Autodesk Fusion 360 part; units mm, degrees
(part 3 of 40)
  spline S12 degree 5 poles (236.3268, 206.0345) (236.3391, 206.0628) (236.3628, 206.1198) (236.396, 206.2062) (236.4359, 206.3229) (236.4798, 206.4711) (236.5193, 206.6208) (236.5561, 206.7714) (236.5915, 206.9226) (236.626, 207.0741) (236.6594, 207.226) (236.6914, 207.3783) (236.7216, 207.5312) (236.7496, 207.6848) (236.7755, 207.8391) (236.7994, 207.994) (236.8217, 208.1494) (236.8425, 208.3052) (236.8621, 208.4614) (236.8805, 208.6179) (236.8978, 208.7747) (236.9138, 208.9318) (236.9285, 209.0893) (236.9418, 209.2471) (236.9538, 209.4053) (236.9645, 209.5638) (236.974, 209.7226) (236.9824, 209.8817) (236.9897, 210.0411) (236.9958, 210.2007) (237.0009, 210.3605) (237.0049, 210.5206) (237.0077, 210.6809) (237.0096, 210.8415) (237.0103, 211.0023) (237.01, 211.1633) (237.0086, 211.3245) (237.0062, 211.4859) (237.0028, 211.6475) (236.9985, 211.8093) (236.9931, 211.9712) (236.9868, 212.1334) (236.9795, 212.2957) (236.9712, 212.4581) (236.962, 212.6207) (236.9519, 212.7835) (236.9408, 212.9464) (236.9287, 213.1095) (236.9158, 213.2727) (236.902, 213.436) (236.8872, 213.5995) (236.8716, 213.7631) (236.855, 213.9268) (236.8376, 214.0906) (236.8193, 214.2545) (236.8001, 214.4185) (236.78, 214.5826) (236.7591, 214.7468) (236.7374, 214.9111) (236.7148, 215.0755) (236.6913, 215.24) (236.667, 215.4046) (236.6418, 215.5692) (236.6159, 215.734) (236.5891, 215.8987) (236.5614, 216.0636) (236.533, 216.2285) (236.5038, 216.3935) (236.4737, 216.5585) (236.4428, 216.7236) (236.4112, 216.8887) (236.3852, 217.0208) (236.3654, 217.1199) (236.352, 217.186) (236.3452, 217.2191) knots 0 0 0 0 0 0 0.01428571 0.02857143 0.04285714 0.05714286 0.07142857 0.08571429 0.1 0.11428571 0.12857143 0.14285714 0.15714286 0.17142857 0.18571429 0.2 0.21428571 0.22857143 0.24285714 0.25714286 0.27142857 0.28571429 0.3 0.31428571 0.32857143 0.34285714 0.35714286 0.37142857 0.38571429 0.4 0.41428571 0.42857143 0.44285714 0.45714286 0.47142857 0.48571429 0.5 0.51428571 0.52857143 0.54285714 0.55714286 0.57142857 0.58571429 0.6 0.61428571 0.62857143 0.64285714 0.65714286 0.67142857 0.68571429 0.7 0.71428571 0.72857143 0.74285714 0.75714286 0.77142857 0.78571429 0.8 0.81428571 0.82857143 0.84285714 0.85714286 0.87142857 0.88571429 0.9 0.91428571 0.92857143 0.94285714 0.95714286 0.97142857 0.98571429 1 1 1 1 1 1
  line L899 (236.3268, 206.0345) -> (236.3391, 206.0628) construction
  line L900 (236.3391, 206.0628) -> (236.3628, 206.1198) construction
  line L901 (236.3628, 206.1198) -> (236.396, 206.2062) construction
  line L902 (236.396, 206.2062) -> (236.4359, 206.3229) construction
  line L903 (236.4359, 206.3229) -> (236.4798, 206.4711) construction
  line L904 (236.4798, 206.4711) -> (236.5193, 206.6208) construction
  line L905 (236.5193, 206.6208) -> (236.5561, 206.7714) construction
  line L906 (236.5561, 206.7714) -> (236.5915, 206.9226) construction
  line L907 (236.5915, 206.9226) -> (236.626, 207.0741) construction
  line L908 (236.626, 207.0741) -> (236.6594, 207.226) construction
  line L909 (236.6594, 207.226) -> (236.6914, 207.3783) construction
  line L910 (236.6914, 207.3783) -> (236.7216, 207.5312) construction
  line L911 (236.7216, 207.5312) -> (236.7496, 207.6848) construction
  line L912 (236.7496, 207.6848) -> (236.7755, 207.8391) construction
  line L913 (236.7755, 207.8391) -> (236.7994, 207.994) construction
  line L914 (236.7994, 207.994) -> (236.8217, 208.1494) construction
  line L915 (236.8217, 208.1494) -> (236.8425, 208.3052) construction
  line L916 (236.8425, 208.3052) -> (236.8621, 208.4614) construction
  line L917 (236.8621, 208.4614) -> (236.8805, 208.6179) construction
  line L918 (236.8805, 208.6179) -> (236.8978, 208.7747) construction
  line L919 (236.8978, 208.7747) -> (236.9138, 208.9318) construction
  line L920 (236.9138, 208.9318) -> (236.9285, 209.0893) construction
  line L921 (236.9285, 209.0893) -> (236.9418, 209.2471) construction
  line L922 (236.9418, 209.2471) -> (236.9538, 209.4053) construction
  line L923 (236.9538, 209.4053) -> (236.9645, 209.5638) construction
  line L924 (236.9645, 209.5638) -> (236.974, 209.7226) construction
  line L925 (236.974, 209.7226) -> (236.9824, 209.8817) construction
  line L926 (236.9824, 209.8817) -> (236.9897, 210.0411) construction
  line L927 (236.9897, 210.0411) -> (236.9958, 210.2007) construction
  line L928 (236.9958, 210.2007) -> (237.0009, 210.3605) construction
  line L929 (237.0009, 210.3605) -> (237.0049, 210.5206) construction
  line L930 (237.0049, 210.5206) -> (237.0077, 210.6809) construction
  line L931 (237.0077, 210.6809) -> (237.0096, 210.8415) construction
  line L932 (237.0096, 210.8415) -> (237.0103, 211.0023) construction
  line L933 (237.0103, 211.0023) -> (237.01, 211.1633) construction
  line L934 (237.01, 211.1633) -> (237.0086, 211.3245) construction
  line L935 (237.0086, 211.3245) -> (237.0062, 211.4859) construction
  line L936 (237.0062, 211.4859) -> (237.0028, 211.6475) construction
  line L937 (237.0028, 211.6475) -> (236.9985, 211.8093) construction
  line L938 (236.9985, 211.8093) -> (236.9931, 211.9712) construction
  line L939 (236.9931, 211.9712) -> (236.9868, 212.1334) construction
  line L940 (236.9868, 212.1334) -> (236.9795, 212.2957) construction
  line L941 (236.9795, 212.2957) -> (236.9712, 212.4581) construction
  line L942 (236.9712, 212.4581) -> (236.962, 212.6207) construction
  line L943 (236.962, 212.6207) -> (236.9519, 212.7835) construction
  line L944 (236.9519, 212.7835) -> (236.9408, 212.9464) construction
  line L945 (236.9408, 212.9464) -> (236.9287, 213.1095) construction
  line L946 (236.9287, 213.1095) -> (236.9158, 213.2727) construction
  line L947 (236.9158, 213.2727) -> (236.902, 213.436) construction
  line L948 (236.902, 213.436) -> (236.8872, 213.5995) construction
  line L949 (236.8872, 213.5995) -> (236.8716, 213.7631) construction
  line L950 (236.8716, 213.7631) -> (236.855, 213.9268) construction
  line L951 (236.855, 213.9268) -> (236.8376, 214.0906) construction
  line L952 (236.8376, 214.0906) -> (236.8193, 214.2545) construction
  line L953 (236.8193, 214.2545) -> (236.8001, 214.4185) construction
  line L954 (236.8001, 214.4185) -> (236.78, 214.5826) construction
  line L955 (236.78, 214.5826) -> (236.7591, 214.7468) construction
  line L956 (236.7591, 214.7468) -> (236.7374, 214.9111) construction
  line L957 (236.7374, 214.9111) -> (236.7148, 215.0755) construction
  line L958 (236.7148, 215.0755) -> (236.6913, 215.24) construction
  line L959 (236.6913, 215.24) -> (236.667, 215.4046) construction
  line L960 (236.667, 215.4046) -> (236.6418, 215.5692) construction
  line L961 (236.6418, 215.5692) -> (236.6159, 215.734) construction
  line L962 (236.6159, 215.734) -> (236.5891, 215.8987) construction
  line L963 (236.5891, 215.8987) -> (236.5614, 216.0636) construction
  line L964 (236.5614, 216.0636) -> (236.533, 216.2285) construction
  line L965 (236.533, 216.2285) -> (236.5038, 216.3935) construction
  line L966 (236.5038, 216.3935) -> (236.4737, 216.5585) construction
  line L967 (236.4737, 216.5585) -> (236.4428, 216.7236) construction
  line L968 (236.4428, 216.7236) -> (236.4112, 216.8887) construction
  line L969 (236.4112, 216.8887) -> (236.3852, 217.0208) construction
  line L970 (236.3852, 217.0208) -> (236.3654, 217.1199) construction
  line L971 (236.3654, 217.1199) -> (236.352, 217.186) construction
  line L972 (236.352, 217.186) -> (236.3452, 217.2191) construction
  spline S13 degree 5 poles (236.3268, 206.0345) (236.3391, 206.0628) (236.3628, 206.1198) (236.396, 206.2062) (236.4359, 206.3229) (236.4798, 206.4711) (236.5193, 206.6208) (236.5561, 206.7714) (236.5915, 206.9226) (236.626, 207.0741) (236.6594, 207.226) (236.6914, 207.3783) (236.7216, 207.5312) (236.7496, 207.6848) (236.7755, 207.8391) (236.7994, 207.994) (236.8217, 208.1494) (236.8425, 208.3052) (236.8621, 208.4614) (236.8805, 208.6179) (236.8978, 208.7747) (236.9138, 208.9318) (236.9285, 209.0893) (236.9418, 209.2471) (236.9538, 209.4053) (236.9645, 209.5638) (236.974, 209.7226) (236.9824, 209.8817) (236.9897, 210.0411) (236.9958, 210.2007) (237.0009, 210.3605) (237.0049, 210.5206) (237.0077, 210.6809) (237.0096, 210.8415) (237.0103, 211.0023) (237.01, 211.1633) (237.0086, 211.3245) (237.0062, 211.4859) (237.0028, 211.6475) (236.9985, 211.8093) (236.9931, 211.9712) (236.9868, 212.1334) (236.9795, 212.2957) (236.9712, 212.4581) (236.962, 212.6207) (236.9519, 212.7835) (236.9408, 212.9464) (236.9287, 213.1095) (236.9158, 213.2727) (236.902, 213.436) (236.8872, 213.5995) (236.8716, 213.7631) (236.855, 213.9268) (236.8376, 214.0906) (236.8193, 214.2545) (236.8001, 214.4185) (236.78, 214.5826) (236.7591, 214.7468) (236.7374, 214.9111) (236.7148, 215.0755) (236.6913, 215.24) (236.667, 215.4046) (236.6418, 215.5692) (236.6159, 215.734) (236.5891, 215.8987) (236.5614, 216.0636) (236.533, 216.2285) (236.5038, 216.3935) (236.4737, 216.5585) (236.4428, 216.7236) (236.4112, 216.8887) (236.3852, 217.0208) (236.3654, 217.1199) (236.352, 217.186) (236.3452, 217.2191) knots 0 0 0 0 0 0 0.01428571 0.02857143 0.04285714 0.05714286 0.07142857 0.08571429 0.1 0.11428571 0.12857143 0.14285714 0.15714286 0.17142857 0.18571429 0.2 0.21428571 0.22857143 0.24285714 0.25714286 0.27142857 0.28571429 0.3 0.31428571 0.32857143 0.34285714 0.35714286 0.37142857 0.38571429 0.4 0.41428571 0.42857143 0.44285714 0.45714286 0.47142857 0.48571429 0.5 0.51428571 0.52857143 0.54285714 0.55714286 0.57142857 0.58571429 0.6 0.61428571 0.62857143 0.64285714 0.65714286 0.67142857 0.68571429 0.7 0.71428571 0.72857143 0.74285714 0.75714286 0.77142857 0.78571429 0.8 0.81428571 0.82857143 0.84285714 0.85714286 0.87142857 0.88571429 0.9 0.91428571 0.92857143 0.94285714 0.95714286 0.97142857 0.98571429 1 1 1 1 1 1
  line L973 (236.3268, 206.0345) -> (236.3391, 206.0628) construction
  line L974 (236.3391, 206.0628) -> (236.3628, 206.1198) construction
  line L975 (236.3628, 206.1198) -> (236.396, 206.2062) construction
  line L976 (236.396, 206.2062) -> (236.4359, 206.3229) construction
  line L977 (236.4359, 206.3229) -> (236.4798, 206.4711) construction
  line L978 (236.4798, 206.4711) -> (236.5193, 206.6208) construction
  line L979 (236.5193, 206.6208) -> (236.5561, 206.7714) construction
  line L980 (236.5561, 206.7714) -> (236.5915, 206.9226) construction
  line L981 (236.5915, 206.9226) -> (236.626, 207.0741) construction
  line L982 (236.626, 207.0741) -> (236.6594, 207.226) construction
  line L983 (236.6594, 207.226) -> (236.6914, 207.3783) construction
  line L984 (236.6914, 207.3783) -> (236.7216, 207.5312) construction
  line L985 (236.7216, 207.5312) -> (236.7496, 207.6848) construction
  line L986 (236.7496, 207.6848) -> (236.7755, 207.8391) construction
  line L987 (236.7755, 207.8391) -> (236.7994, 207.994) construction
  line L988 (236.7994, 207.994) -> (236.8217, 208.1494) construction
  line L989 (236.8217, 208.1494) -> (236.8425, 208.3052) construction
  line L990 (236.8425, 208.3052) -> (236.8621, 208.4614) construction
  line L991 (236.8621, 208.4614) -> (236.8805, 208.6179) construction
  line L992 (236.8805, 208.6179) -> (236.8978, 208.7747) construction
  line L993 (236.8978, 208.7747) -> (236.9138, 208.9318) construction
  line L994 (236.9138, 208.9318) -> (236.9285, 209.0893) construction
  line L995 (236.9285, 209.0893) -> (236.9418, 209.2471) construction
  line L996 (236.9418, 209.2471) -> (236.9538, 209.4053) construction
  line L997 (236.9538, 209.4053) -> (236.9645, 209.5638) construction
  line L998 (236.9645, 209.5638) -> (236.974, 209.7226) construction
  line L999 (236.974, 209.7226) -> (236.9824, 209.8817) construction
  line L1000 (236.9824, 209.8817) -> (236.9897, 210.0411) construction
  line L1001 (236.9897, 210.0411) -> (236.9958, 210.2007) construction
  line L1002 (236.9958, 210.2007) -> (237.0009, 210.3605) construction
  line L1003 (237.0009, 210.3605) -> (237.0049, 210.5206) construction
  line L1004 (237.0049, 210.5206) -> (237.0077, 210.6809) construction
  line L1005 (237.0077, 210.6809) -> (237.0096, 210.8415) construction
  line L1006 (237.0096, 210.8415) -> (237.0103, 211.0023) construction
  line L1007 (237.0103, 211.0023) -> (237.01, 211.1633) construction
  line L1008 (237.01, 211.1633) -> (237.0086, 211.3245) construction
  line L1009 (237.0086, 211.3245) -> (237.0062, 211.4859) construction
  line L1010 (237.0062, 211.4859) -> (237.0028, 211.6475) construction
  line L1011 (237.0028, 211.6475) -> (236.9985, 211.8093) construction
  line L1012 (236.9985, 211.8093) -> (236.9931, 211.9712) construction
  line L1013 (236.9931, 211.9712) -> (236.9868, 212.1334) construction
  line L1014 (236.9868, 212.1334) -> (236.9795, 212.2957) construction
  line L1015 (236.9795, 212.2957) -> (236.9712, 212.4581) construction
  line L1016 (236.9712, 212.4581) -> (236.962, 212.6207) construction
  line L1017 (236.962, 212.6207) -> (236.9519, 212.7835) construction
  line L1018 (236.9519, 212.7835) -> (236.9408, 212.9464) construction
  line L1019 (236.9408, 212.9464) -> (236.9287, 213.1095) construction
  line L1020 (236.9287, 213.1095) -> (236.9158, 213.2727) construction
  line L1021 (236.9158, 213.2727) -> (236.902, 213.436) construction
  line L1022 (236.902, 213.436) -> (236.8872, 213.5995) construction
  line L1023 (236.8872, 213.5995) -> (236.8716, 213.7631) construction
  line L1024 (236.8716, 213.7631) -> (236.855, 213.9268) construction
  line L1025 (236.855, 213.9268) -> (236.8376, 214.0906) construction
  line L1026 (236.8376, 214.0906) -> (236.8193, 214.2545) construction
  line L1027 (236.8193, 214.2545) -> (236.8001, 214.4185) construction
  line L1028 (236.8001, 214.4185) -> (236.78, 214.5826) construction
  line L1029 (236.78, 214.5826) -> (236.7591, 214.7468) construction
  line L1030 (236.7591, 214.7468) -> (236.7374, 214.9111) construction
  line L1031 (236.7374, 214.9111) -> (236.7148, 215.0755) construction
  line L1032 (236.7148, 215.0755) -> (236.6913, 215.24) construction
  line L1033 (236.6913, 215.24) -> (236.667, 215.4046) construction
  line L1034 (236.667, 215.4046) -> (236.6418, 215.5692) construction
  line L1035 (236.6418, 215.5692) -> (236.6159, 215.734) construction
  line L1036 (236.6159, 215.734) -> (236.5891, 215.8987) construction
  line L1037 (236.5891, 215.8987) -> (236.5614, 216.0636) construction
  line L1038 (236.5614, 216.0636) -> (236.533, 216.2285) construction
  line L1039 (236.533, 216.2285) -> (236.5038, 216.3935) construction
  line L1040 (236.5038, 216.3935) -> (236.4737, 216.5585) construction
  line L1041 (236.4737, 216.5585) -> (236.4428, 216.7236) construction
  line L1042 (236.4428, 216.7236) -> (236.4112, 216.8887) construction
  line L1043 (236.4112, 216.8887) -> (236.3852, 217.0208) construction
  line L1044 (236.3852, 217.0208) -> (236.3654, 217.1199) construction
  line L1045 (236.3654, 217.1199) -> (236.352, 217.186) construction
  line L1046 (236.352, 217.186) -> (236.3452, 217.2191) construction
  line L1047 (167.5414, 110.7517) -> (166.3167, 109.6737)
  line L1048 (167.5414, 110.7517) -> (166.3167, 109.6737)
  arc A19 (235.6801, 204.5366) -> (236.6621, 201.9354) centre (237.5162, 203.7438) ccw
  line L1049 (235.6801, 204.5366) -> (236.3268, 206.0345)
  line L1050 (235.6801, 204.5366) -> (236.3268, 206.0345)
  arc A20 (235.6801, 204.5366) -> (236.6621, 201.9354) centre (237.5162, 203.7438) ccw
  line L1051 (167.5414, 189.2483) -> (166.3167, 190.3263)
  spline S14 degree 5 poles (243.2435, 202.5103) (243.2592, 202.5368) (243.2914, 202.5895) (243.3417, 202.6672) (243.4127, 202.7681) (243.5068, 202.8906) (243.6047, 203.0106) (243.7049, 203.1289) (243.8064, 203.2464) (243.9087, 203.3634) (244.012, 203.4797) (244.1164, 203.5951) (244.2223, 203.7094) (244.3301, 203.8224) (244.4397, 203.934) (244.551, 204.0444) (244.6636, 204.1537) (244.7775, 204.2622) (244.8923, 204.3698) (245.008, 204.4767) (245.1247, 204.5828) (245.2425, 204.6881) (245.3612, 204.7926) (245.4811, 204.8961) (245.602, 204.9988) (245.7239, 205.1007) (245.8468, 205.2017) (245.9706, 205.302) (246.0953, 205.4015) (246.2208, 205.5003) (246.3471, 205.5984) (246.4743, 205.6957) (246.6023, 205.7923) (246.7311, 205.8881) (246.8608, 205.9832) (246.9912, 206.0776) (247.1225, 206.1712) (247.2544, 206.2642) (247.3872, 206.3564) (247.5206, 206.448) (247.6548, 206.5388) (247.7897, 206.629) (247.9253, 206.7185) (248.0615, 206.8073) (248.1985, 206.8955) (248.3362, 206.9829) (248.4745, 207.0697) (248.6135, 207.1558) (248.7531, 207.2413) (248.8934, 207.3261) (249.0343, 207.4102) (249.1758, 207.4937) (249.318, 207.5765) (249.4608, 207.6587) (249.6041, 207.7403) (249.7481, 207.8212) (249.8927, 207.9014) (250.0378, 207.981) (250.1835, 208.06) (250.3298, 208.1383) (250.4767, 208.216) (250.6241, 208.2931) (250.7721, 208.3695) (250.9206, 208.4453) (251.0697, 208.5205) (251.2193, 208.595) (251.3694, 208.669) (251.5201, 208.7423) (251.6713, 208.8149) (251.8229, 208.887) (251.9751, 208.9584) (252.0973, 209.0151) (252.1892, 209.0573) (252.2505, 209.0853) (252.2812, 209.0993) knots 0 0 0 0 0 0 0.01428571 0.02857143 0.04285714 0.05714286 0.07142857 0.08571429 0.1 0.11428571 0.12857143 0.14285714 0.15714286 0.17142857 0.18571429 0.2 0.21428571 0.22857143 0.24285714 0.25714286 0.27142857 0.28571429 0.3 0.31428571 0.32857143 0.34285714 0.35714286 0.37142857 0.38571429 0.4 0.41428571 0.42857143 0.44285714 0.45714286 0.47142857 0.48571429 0.5 0.51428571 0.52857143 0.54285714 0.55714286 0.57142857 0.58571429 0.6 0.61428571 0.62857143 0.64285714 0.65714286 0.67142857 0.68571429 0.7 0.71428571 0.72857143 0.74285714 0.75714286 0.77142857 0.78571429 0.8 0.81428571 0.82857143 0.84285714 0.85714286 0.87142857 0.88571429 0.9 0.91428571 0.92857143 0.94285714 0.95714286 0.97142857 0.98571429 1 1 1 1 1 1
  line L1052 (243.2435, 202.5103) -> (243.2592, 202.5368) construction
  line L1053 (243.2592, 202.5368) -> (243.2914, 202.5895) construction
  line L1054 (243.2914, 202.5895) -> (243.3417, 202.6672) construction
  line L1055 (243.3417, 202.6672) -> (243.4127, 202.7681) construction
  line L1056 (243.4127, 202.7681) -> (243.5068, 202.8906) construction
  line L1057 (243.5068, 202.8906) -> (243.6047, 203.0106) construction
  line L1058 (243.6047, 203.0106) -> (243.7049, 203.1289) construction
  line L1059 (243.7049, 203.1289) -> (243.8064, 203.2464) construction
  line L1060 (243.8064, 203.2464) -> (243.9087, 203.3634) construction
  line L1061 (243.9087, 203.3634) -> (244.012, 203.4797) construction
  line L1062 (244.012, 203.4797) -> (244.1164, 203.5951) construction
  line L1063 (244.1164, 203.5951) -> (244.2223, 203.7094) construction
  line L1064 (244.2223, 203.7094) -> (244.3301, 203.8224) construction
  line L1065 (244.3301, 203.8224) -> (244.4397, 203.934) construction
  line L1066 (244.4397, 203.934) -> (244.551, 204.0444) construction
  line L1067 (244.551, 204.0444) -> (244.6636, 204.1537) construction
  line L1068 (244.6636, 204.1537) -> (244.7775, 204.2622) construction
  line L1069 (244.7775, 204.2622) -> (244.8923, 204.3698) construction
  line L1070 (244.8923, 204.3698) -> (245.008, 204.4767) construction
  line L1071 (245.008, 204.4767) -> (245.1247, 204.5828) construction
  line L1072 (245.1247, 204.5828) -> (245.2425, 204.6881) construction
  line L1073 (245.2425, 204.6881) -> (245.3612, 204.7926) construction
  line L1074 (245.3612, 204.7926) -> (245.4811, 204.8961) construction
  line L1075 (245.4811, 204.8961) -> (245.602, 204.9988) construction
  line L1076 (245.602, 204.9988) -> (245.7239, 205.1007) construction
  line L1077 (245.7239, 205.1007) -> (245.8468, 205.2017) construction
  line L1078 (245.8468, 205.2017) -> (245.9706, 205.302) construction
  line L1079 (245.9706, 205.302) -> (246.0953, 205.4015) construction
  line L1080 (246.0953, 205.4015) -> (246.2208, 205.5003) construction
  line L1081 (246.2208, 205.5003) -> (246.3471, 205.5984) construction
  line L1082 (246.3471, 205.5984) -> (246.4743, 205.6957) construction
  line L1083 (246.4743, 205.6957) -> (246.6023, 205.7923) construction
  line L1084 (246.6023, 205.7923) -> (246.7311, 205.8881) construction
  line L1085 (246.7311, 205.8881) -> (246.8608, 205.9832) construction
  line L1086 (246.8608, 205.9832) -> (246.9912, 206.0776) construction
  line L1087 (246.9912, 206.0776) -> (247.1225, 206.1712) construction
  line L1088 (247.1225, 206.1712) -> (247.2544, 206.2642) construction
  line L1089 (247.2544, 206.2642) -> (247.3872, 206.3564) construction
  line L1090 (247.3872, 206.3564) -> (247.5206, 206.448) construction
  line L1091 (247.5206, 206.448) -> (247.6548, 206.5388) construction
  line L1092 (247.6548, 206.5388) -> (247.7897, 206.629) construction
  line L1093 (247.7897, 206.629) -> (247.9253, 206.7185) construction
  line L1094 (247.9253, 206.7185) -> (248.0615, 206.8073) construction
  line L1095 (248.0615, 206.8073) -> (248.1985, 206.8955) construction
  line L1096 (248.1985, 206.8955) -> (248.3362, 206.9829) construction
  line L1097 (248.3362, 206.9829) -> (248.4745, 207.0697) construction
  line L1098 (248.4745, 207.0697) -> (248.6135, 207.1558) construction
  line L1099 (248.6135, 207.1558) -> (248.7531, 207.2413) construction
  line L1100 (248.7531, 207.2413) -> (248.8934, 207.3261) construction
  line L1101 (248.8934, 207.3261) -> (249.0343, 207.4102) construction
  line L1102 (249.0343, 207.4102) -> (249.1758, 207.4937) construction
  line L1103 (249.1758, 207.4937) -> (249.318, 207.5765) construction
  line L1104 (249.318, 207.5765) -> (249.4608, 207.6587) construction
  line L1105 (249.4608, 207.6587) -> (249.6041, 207.7403) construction
  line L1106 (249.6041, 207.7403) -> (249.7481, 207.8212) construction
  line L1107 (249.7481, 207.8212) -> (249.8927, 207.9014) construction
  line L1108 (249.8927, 207.9014) -> (250.0378, 207.981) construction
  line L1109 (250.0378, 207.981) -> (250.1835, 208.06) construction
  line L1110 (250.1835, 208.06) -> (250.3298, 208.1383) construction
  line L1111 (250.3298, 208.1383) -> (250.4767, 208.216) construction
  line L1112 (250.4767, 208.216) -> (250.6241, 208.2931) construction
  line L1113 (250.6241, 208.2931) -> (250.7721, 208.3695) construction
  line L1114 (250.7721, 208.3695) -> (250.9206, 208.4453) construction
  line L1115 (250.9206, 208.4453) -> (251.0697, 208.5205) construction
  line L1116 (251.0697, 208.5205) -> (251.2193, 208.595) construction
  line L1117 (251.2193, 208.595) -> (251.3694, 208.669) construction
  line L1118 (251.3694, 208.669) -> (251.5201, 208.7423) construction
  line L1119 (251.5201, 208.7423) -> (251.6713, 208.8149) construction
  line L1120 (251.6713, 208.8149) -> (251.8229, 208.887) construction
  line L1121 (251.8229, 208.887) -> (251.9751, 208.9584) construction
  line L1122 (251.9751, 208.9584) -> (252.0973, 209.0151) construction
  line L1123 (252.0973, 209.0151) -> (252.1892, 209.0573) construction
  line L1124 (252.1892, 209.0573) -> (252.2505, 209.0853) construction
  line L1125 (252.2505, 209.0853) -> (252.2812, 209.0993) construction
  spline S15 degree 5 poles (243.2435, 202.5103) (243.2592, 202.5368) (243.2914, 202.5895) (243.3417, 202.6672) (243.4127, 202.7681) (243.5068, 202.8906) (243.6047, 203.0106) (243.7049, 203.1289) (243.8064, 203.2464) (243.9087, 203.3634) (244.012, 203.4797) (244.1164, 203.5951) (244.2223, 203.7094) (244.3301, 203.8224) (244.4397, 203.934) (244.551, 204.0444) (244.6636, 204.1537) (244.7775, 204.2622) (244.8923, 204.3698) (245.008, 204.4767) (245.1247, 204.5828) (245.2425, 204.6881) (245.3612, 204.7926) (245.4811, 204.8961) (245.602, 204.9988) (245.7239, 205.1007) (245.8468, 205.2017) (245.9706, 205.302) (246.0953, 205.4015) (246.2208, 205.5003) (246.3471, 205.5984) (246.4743, 205.6957) (246.6023, 205.7923) (246.7311, 205.8881) (246.8608, 205.9832) (246.9912, 206.0776) (247.1225, 206.1712) (247.2544, 206.2642) (247.3872, 206.3564) (247.5206, 206.448) (247.6548, 206.5388) (247.7897, 206.629) (247.9253, 206.7185) (248.0615, 206.8073) (248.1985, 206.8955) (248.3362, 206.9829) (248.4745, 207.0697) (248.6135, 207.1558) (248.7531, 207.2413) (248.8934, 207.3261) (249.0343, 207.4102) (249.1758, 207.4937) (249.318, 207.5765) (249.4608, 207.6587) (249.6041, 207.7403) (249.7481, 207.8212) (249.8927, 207.9014) (250.0378, 207.981) (250.1835, 208.06) (250.3298, 208.1383) (250.4767, 208.216) (250.6241, 208.2931) (250.7721, 208.3695) (250.9206, 208.4453) (251.0697, 208.5205) (251.2193, 208.595) (251.3694, 208.669) (251.5201, 208.7423) (251.6713, 208.8149) (251.8229, 208.887) (251.9751, 208.9584) (252.0973, 209.0151) (252.1892, 209.0573) (252.2505, 209.0853) (252.2812, 209.0993) knots 0 0 0 0 0 0 0.01428571 0.02857143 0.04285714 0.05714286 0.07142857 0.08571429 0.1 0.11428571 0.12857143 0.14285714 0.15714286 0.17142857 0.18571429 0.2 0.21428571 0.22857143 0.24285714 0.25714286 0.27142857 0.28571429 0.3 0.31428571 0.32857143 0.34285714 0.35714286 0.37142857 0.38571429 0.4 0.41428571 0.42857143 0.44285714 0.45714286 0.47142857 0.48571429 0.5 0.51428571 0.52857143 0.54285714 0.55714286 0.57142857 0.58571429 0.6 0.61428571 0.62857143 0.64285714 0.65714286 0.67142857 0.68571429 0.7 0.71428571 0.72857143 0.74285714 0.75714286 0.77142857 0.78571429 0.8 0.81428571 0.82857143 0.84285714 0.85714286 0.87142857 0.88571429 0.9 0.91428571 0.92857143 0.94285714 0.95714286 0.97142857 0.98571429 1 1 1 1 1 1
  line L1126 (243.2435, 202.5103) -> (243.2592, 202.5368) construction
  line L1127 (243.2592, 202.5368) -> (243.2914, 202.5895) construction
  line L1128 (243.2914, 202.5895) -> (243.3417, 202.6672) construction
  line L1129 (243.3417, 202.6672) -> (243.4127, 202.7681) construction
  line L1130 (243.4127, 202.7681) -> (243.5068, 202.8906) construction
  line L1131 (243.5068, 202.8906) -> (243.6047, 203.0106) construction
  line L1132 (243.6047, 203.0106) -> (243.7049, 203.1289) construction
  line L1133 (243.7049, 203.1289) -> (243.8064, 203.2464) construction
  line L1134 (243.8064, 203.2464) -> (243.9087, 203.3634) construction
  line L1135 (243.9087, 203.3634) -> (244.012, 203.4797) construction
  line L1136 (244.012, 203.4797) -> (244.1164, 203.5951) construction
  line L1137 (244.1164, 203.5951) -> (244.2223, 203.7094) construction
  line L1138 (244.2223, 203.7094) -> (244.3301, 203.8224) construction
  line L1139 (244.3301, 203.8224) -> (244.4397, 203.934) construction
  line L1140 (244.4397, 203.934) -> (244.551, 204.0444) construction
  line L1141 (244.551, 204.0444) -> (244.6636, 204.1537) construction
  line L1142 (244.6636, 204.1537) -> (244.7775, 204.2622) construction
  line L1143 (244.7775, 204.2622) -> (244.8923, 204.3698) construction
  line L1144 (244.8923, 204.3698) -> (245.008, 204.4767) construction
  line L1145 (245.008, 204.4767) -> (245.1247, 204.5828) construction
  line L1146 (245.1247, 204.5828) -> (245.2425, 204.6881) construction
  line L1147 (245.2425, 204.6881) -> (245.3612, 204.7926) construction
  line L1148 (245.3612, 204.7926) -> (245.4811, 204.8961) construction
  line L1149 (245.4811, 204.8961) -> (245.602, 204.9988) construction
  line L1150 (245.602, 204.9988) -> (245.7239, 205.1007) construction
  line L1151 (245.7239, 205.1007) -> (245.8468, 205.2017) construction
  line L1152 (245.8468, 205.2017) -> (245.9706, 205.302) construction
  line L1153 (245.9706, 205.302) -> (246.0953, 205.4015) construction
  line L1154 (246.0953, 205.4015) -> (246.2208, 205.5003) construction
  line L1155 (246.2208, 205.5003) -> (246.3471, 205.5984) construction
  line L1156 (246.3471, 205.5984) -> (246.4743, 205.6957) construction
  line L1157 (246.4743, 205.6957) -> (246.6023, 205.7923) construction
  line L1158 (246.6023, 205.7923) -> (246.7311, 205.8881) construction
  line L1159 (246.7311, 205.8881) -> (246.8608, 205.9832) construction
  line L1160 (246.8608, 205.9832) -> (246.9912, 206.0776) construction
  line L1161 (246.9912, 206.0776) -> (247.1225, 206.1712) construction
  line L1162 (247.1225, 206.1712) -> (247.2544, 206.2642) construction
  line L1163 (247.2544, 206.2642) -> (247.3872, 206.3564) construction
  line L1164 (247.3872, 206.3564) -> (247.5206, 206.448) construction
  line L1165 (247.5206, 206.448) -> (247.6548, 206.5388) construction
  line L1166 (247.6548, 206.5388) -> (247.7897, 206.629) construction
  line L1167 (247.7897, 206.629) -> (247.9253, 206.7185) construction
  line L1168 (247.9253, 206.7185) -> (248.0615, 206.8073) construction
  line L1169 (248.0615, 206.8073) -> (248.1985, 206.8955) construction
  line L1170 (248.1985, 206.8955) -> (248.3362, 206.9829) construction
  line L1171 (248.3362, 206.9829) -> (248.4745, 207.0697) construction
  line L1172 (248.4745, 207.0697) -> (248.6135, 207.1558) construction
  line L1173 (248.6135, 207.1558) -> (248.7531, 207.2413) construction
  line L1174 (248.7531, 207.2413) -> (248.8934, 207.3261) construction
  line L1175 (248.8934, 207.3261) -> (249.0343, 207.4102) construction
  line L1176 (249.0343, 207.4102) -> (249.1758, 207.4937) construction
  line L1177 (249.1758, 207.4937) -> (249.318, 207.5765) construction
  line L1178 (249.318, 207.5765) -> (249.4608, 207.6587) construction
  line L1179 (249.4608, 207.6587) -> (249.6041, 207.7403) construction
  line L1180 (249.6041, 207.7403) -> (249.7481, 207.8212) construction
  line L1181 (249.7481, 207.8212) -> (249.8927, 207.9014) construction
  line L1182 (249.8927, 207.9014) -> (250.0378, 207.981) construction
  line L1183 (250.0378, 207.981) -> (250.1835, 208.06) construction
  line L1184 (250.1835, 208.06) -> (250.3298, 208.1383) construction
  line L1185 (250.3298, 208.1383) -> (250.4767, 208.216) construction
  line L1186 (250.4767, 208.216) -> (250.6241, 208.2931) construction
  line L1187 (250.6241, 208.2931) -> (250.7721, 208.3695) construction
  line L1188 (250.7721, 208.3695) -> (250.9206, 208.4453) construction
  line L1189 (250.9206, 208.4453) -> (251.0697, 208.5205) construction
  line L1190 (251.0697, 208.5205) -> (251.2193, 208.595) construction
  line L1191 (251.2193, 208.595) -> (251.3694, 208.669) construction
  line L1192 (251.3694, 208.669) -> (251.5201, 208.7423) construction
  line L1193 (251.5201, 208.7423) -> (251.6713, 208.8149) construction
  line L1194 (251.6713, 208.8149) -> (251.8229, 208.887) construction
  line L1195 (251.8229, 208.887) -> (251.9751, 208.9584) construction
  line L1196 (251.9751, 208.9584) -> (252.0973, 209.0151) construction
  line L1197 (252.0973, 209.0151) -> (252.1892, 209.0573) construction
  line L1198 (252.1892, 209.0573) -> (252.2505, 209.0853) construction
  line L1199 (252.2505, 209.0853) -> (252.2812, 209.0993) construction
  line L1200 (167.5414, 189.2483) -> (166.3167, 190.3263)
  arc A21 (251.3803, 194.5906) -> (251.5104, 191.8132) centre (252.8816, 193.2692) ccw
  line L1201 (251.3803, 194.5906) -> (252.4583, 195.8153)
  arc A22 (239.7302, 200.3721) -> (236.6621, 201.9354) centre (212.132, 150) ccw
  arc A23 (239.7302, 200.3721) -> (242.4118, 201.1066) centre (240.6912, 202.1261) ccw
  arc A24 (239.7302, 200.3721) -> (242.4118, 201.1066) centre (240.6912, 202.1261) ccw
  line L1202 (251.3803, 194.5906) -> (252.4583, 195.8153)
  line L1203 (242.4118, 201.1066) -> (243.2435, 202.5103)
  arc A25 (251.3803, 194.5906) -> (251.5104, 191.8132) centre (252.8816, 193.2692) ccw
  line L1204 (242.4118, 201.1066) -> (243.2435, 202.5103)
  arc A26 (239.7302, 200.3721) -> (236.6621, 201.9354) centre (212.132, 150) ccw
  arc A27 (268.567, 139.3184) -> (269.1057, 142.7194) centre (212.132, 150) ccw
  line L1205 (271.2762, 144.4572) -> (272.9005, 144.3049)
  line L1206 (271.2762, 144.4572) -> (272.9005, 144.3049)
  arc A28 (268.567, 139.3184) -> (269.1057, 142.7194) centre (212.132, 150) ccw
  arc A29 (271.2762, 144.4572) -> (269.1057, 142.7194) centre (271.0895, 142.4659) ccw
  arc A30 (271.2762, 144.4572) -> (269.1057, 142.7194) centre (271.0895, 142.4659) ccw
  arc A31 (187.6019, 201.9354) -> (184.5338, 200.3721) centre (212.132, 150) ccw
  arc A32 (181.8522, 201.1066) -> (184.5338, 200.3721) centre (183.5728, 202.1261) ccw
  line L1207 (199.127, 92.0377) -> (198.7698, 90.4458)
  arc A33 (201.4504, 93.565) -> (199.127, 92.0377) centre (201.0785, 91.5999) ccw
  line L1208 (181.8522, 201.1066) -> (181.0205, 202.5103)
  arc A34 (181.8522, 201.1066) -> (184.5338, 200.3721) centre (183.5728, 202.1261) ccw
  arc A35 (187.6019, 201.9354) -> (184.5338, 200.3721) centre (212.132, 150) ccw
  line L1209 (199.127, 92.0377) -> (198.7698, 90.4458)
  line L1210 (181.8522, 201.1066) -> (181.0205, 202.5103)
  arc A36 (201.4504, 93.565) -> (199.127, 92.0377) centre (201.0785, 91.5999) ccw
  line L1211 (217.6748, 90.8558) -> (217.8271, 89.2315)
  arc A37 (219.4126, 93.0263) -> (217.6748, 90.8558) centre (219.6661, 91.0425) ccw
  line L1212 (217.6748, 90.8558) -> (217.8271, 89.2315)
  arc A38 (219.4126, 93.0263) -> (217.6748, 90.8558) centre (219.6661, 91.0425) ccw
  line L1213 (263.2386, 180.2798) -> (264.6423, 181.1115)
  arc A39 (263.2386, 180.2798) -> (262.5041, 177.5982) centre (264.2581, 178.5592) ccw
  arc A40 (263.2386, 180.2798) -> (262.5041, 177.5982) centre (264.2581, 178.5592) ccw
  line L1214 (263.2386, 180.2798) -> (264.6423, 181.1115)
  spline S16 degree 5 poles (264.6423, 181.1115) (264.6688, 181.1272) (264.7215, 181.1594) (264.7992, 181.2097) (264.9001, 181.2807) (265.0226, 181.3748) (265.1426, 181.4727) (265.2609, 181.5729) (265.3784, 181.6744) (265.4954, 181.7767) (265.6117, 181.88) (265.7271, 181.9844) (265.8414, 182.0903) (265.9544, 182.1981) (266.066, 182.3077) (266.1764, 182.419) (266.2857, 182.5316) (266.3942, 182.6455) (266.5018, 182.7603) (266.6087, 182.876) (266.7148, 182.9927) (266.8201, 183.1105) (266.9246, 183.2292) (267.0281, 183.3491) (267.1308, 183.47) (267.2327, 183.5919) (267.3337, 183.7148) (267.434, 183.8386) (267.5335, 183.9633) (267.6323, 184.0888) (267.7304, 184.2151) (267.8277, 184.3423) (267.9243, 184.4703) (268.0201, 184.5991) (268.1152, 184.7288) (268.2096, 184.8592) (268.3032, 184.9905) (268.3962, 185.1224) (268.4884, 185.2552) (268.58, 185.3886) (268.6708, 185.5228) (268.761, 185.6577) (268.8505, 185.7933) (268.9393, 185.9295) (269.0275, 186.0665) (269.1149, 186.2042) (269.2017, 186.3425) (269.2878, 186.4815) (269.3733, 186.6211) (269.4581, 186.7614) (269.5422, 186.9023) (269.6257, 187.0438) (269.7085, 187.186) (269.7907, 187.3288) (269.8723, 187.4721) (269.9532, 187.6161) (270.0334, 187.7607) (270.113, 187.9058) (270.192, 188.0515) (270.2703, 188.1978) (270.348, 188.3447) (270.4251, 188.4921) (270.5015, 188.6401) (270.5773, 188.7886) (270.6525, 188.9377) (270.727, 189.0873) (270.801, 189.2374) (270.8743, 189.3881) (270.9469, 189.5393) (271.019, 189.6909) (271.0904, 189.8431) (271.1471, 189.9653) (271.1893, 190.0572) (271.2173, 190.1185) (271.2313, 190.1492) knots 0 0 0 0 0 0 0.01428571 0.02857143 0.04285714 0.05714286 0.07142857 0.08571429 0.1 0.11428571 0.12857143 0.14285714 0.15714286 0.17142857 0.18571429 0.2 0.21428571 0.22857143 0.24285714 0.25714286 0.27142857 0.28571429 0.3 0.31428571 0.32857143 0.34285714 0.35714286 0.37142857 0.38571429 0.4 0.41428571 0.42857143 0.44285714 0.45714286 0.47142857 0.48571429 0.5 0.51428571 0.52857143 0.54285714 0.55714286 0.57142857 0.58571429 0.6 0.61428571 0.62857143 0.64285714 0.65714286 0.67142857 0.68571429 0.7 0.71428571 0.72857143 0.74285714 0.75714286 0.77142857 0.78571429 0.8 0.81428571 0.82857143 0.84285714 0.85714286 0.87142857 0.88571429 0.9 0.91428571 0.92857143 0.94285714 0.95714286 0.97142857 0.98571429 1 1 1 1 1 1
  line L1215 (264.6423, 181.1115) -> (264.6688, 181.1272) construction
  line L1216 (264.6688, 181.1272) -> (264.7215, 181.1594) construction
  line L1217 (264.7215, 181.1594) -> (264.7992, 181.2097) construction
  line L1218 (264.7992, 181.2097) -> (264.9001, 181.2807) construction
  line L1219 (264.9001, 181.2807) -> (265.0226, 181.3748) construction
  line L1220 (265.0226, 181.3748) -> (265.1426, 181.4727) construction
  line L1221 (265.1426, 181.4727) -> (265.2609, 181.5729) construction
  line L1222 (265.2609, 181.5729) -> (265.3784, 181.6744) construction
  line L1223 (265.3784, 181.6744) -> (265.4954, 181.7767) construction
  line L1224 (265.4954, 181.7767) -> (265.6117, 181.88) construction
  line L1225 (265.6117, 181.88) -> (265.7271, 181.9844) construction
  line L1226 (265.7271, 181.9844) -> (265.8414, 182.0903) construction
  line L1227 (265.8414, 182.0903) -> (265.9544, 182.1981) construction
  line L1228 (265.9544, 182.1981) -> (266.066, 182.3077) construction
  line L1229 (266.066, 182.3077) -> (266.1764, 182.419) construction
  line L1230 (266.1764, 182.419) -> (266.2857, 182.5316) construction
  line L1231 (266.2857, 182.5316) -> (266.3942, 182.6455) construction
  line L1232 (266.3942, 182.6455) -> (266.5018, 182.7603) construction
  line L1233 (266.5018, 182.7603) -> (266.6087, 182.876) construction
  line L1234 (266.6087, 182.876) -> (266.7148, 182.9927) construction
  line L1235 (266.7148, 182.9927) -> (266.8201, 183.1105) construction
  line L1236 (266.8201, 183.1105) -> (266.9246, 183.2292) construction
  line L1237 (266.9246, 183.2292) -> (267.0281, 183.3491) construction
  line L1238 (267.0281, 183.3491) -> (267.1308, 183.47) construction
  line L1239 (267.1308, 183.47) -> (267.2327, 183.5919) construction
  line L1240 (267.2327, 183.5919) -> (267.3337, 183.7148) construction
  line L1241 (267.3337, 183.7148) -> (267.434, 183.8386) construction
  line L1242 (267.434, 183.8386) -> (267.5335, 183.9633) construction
  line L1243 (267.5335, 183.9633) -> (267.6323, 184.0888) construction
  line L1244 (267.6323, 184.0888) -> (267.7304, 184.2151) construction
  line L1245 (267.7304, 184.2151) -> (267.8277, 184.3423) construction
  line L1246 (267.8277, 184.3423) -> (267.9243, 184.4703) construction
  line L1247 (267.9243, 184.4703) -> (268.0201, 184.5991) construction
  line L1248 (268.0201, 184.5991) -> (268.1152, 184.7288) construction
  line L1249 (268.1152, 184.7288) -> (268.2096, 184.8592) construction
  line L1250 (268.2096, 184.8592) -> (268.3032, 184.9905) construction
  line L1251 (268.3032, 184.9905) -> (268.3962, 185.1224) construction
  line L1252 (268.3962, 185.1224) -> (268.4884, 185.2552) construction
  line L1253 (268.4884, 185.2552) -> (268.58, 185.3886) construction
  line L1254 (268.58, 185.3886) -> (268.6708, 185.5228) construction
  line L1255 (268.6708, 185.5228) -> (268.761, 185.6577) construction
  line L1256 (268.761, 185.6577) -> (268.8505, 185.7933) construction
  line L1257 (268.8505, 185.7933) -> (268.9393, 185.9295) construction
  line L1258 (268.9393, 185.9295) -> (269.0275, 186.0665) construction
  line L1259 (269.0275, 186.0665) -> (269.1149, 186.2042) construction
  line L1260 (269.1149, 186.2042) -> (269.2017, 186.3425) construction
  line L1261 (269.2017, 186.3425) -> (269.2878, 186.4815) construction
  line L1262 (269.2878, 186.4815) -> (269.3733, 186.6211) construction
  line L1263 (269.3733, 186.6211) -> (269.4581, 186.7614) construction
  line L1264 (269.4581, 186.7614) -> (269.5422, 186.9023) construction
  line L1265 (269.5422, 186.9023) -> (269.6257, 187.0438) construction
  line L1266 (269.6257, 187.0438) -> (269.7085, 187.186) construction
  line L1267 (269.7085, 187.186) -> (269.7907, 187.3288) construction
  line L1268 (269.7907, 187.3288) -> (269.8723, 187.4721) construction
  line L1269 (269.8723, 187.4721) -> (269.9532, 187.6161) construction
  line L1270 (269.9532, 187.6161) -> (270.0334, 187.7607) construction
  line L1271 (270.0334, 187.7607) -> (270.113, 187.9058) construction
  line L1272 (270.113, 187.9058) -> (270.192, 188.0515) construction
  line L1273 (270.192, 188.0515) -> (270.2703, 188.1978) construction
  line L1274 (270.2703, 188.1978) -> (270.348, 188.3447) construction
  line L1275 (270.348, 188.3447) -> (270.4251, 188.4921) construction
  line L1276 (270.4251, 188.4921) -> (270.5015, 188.6401) construction
  line L1277 (270.5015, 188.6401) -> (270.5773, 188.7886) construction
  line L1278 (270.5773, 188.7886) -> (270.6525, 188.9377) construction
  line L1279 (270.6525, 188.9377) -> (270.727, 189.0873) construction
  line L1280 (270.727, 189.0873) -> (270.801, 189.2374) construction
  line L1281 (270.801, 189.2374) -> (270.8743, 189.3881) construction
  line L1282 (270.8743, 189.3881) -> (270.9469, 189.5393) construction
  line L1283 (270.9469, 189.5393) -> (271.019, 189.6909) construction
  line L1284 (271.019, 189.6909) -> (271.0904, 189.8431) construction
  line L1285 (271.0904, 189.8431) -> (271.1471, 189.9653) construction
  line L1286 (271.1471, 189.9653) -> (271.1893, 190.0572) construction
  line L1287 (271.1893, 190.0572) -> (271.2173, 190.1185) construction
  line L1288 (271.2173, 190.1185) -> (271.2313, 190.1492) construction
  spline S17 degree 5 poles (264.6423, 181.1115) (264.6688, 181.1272) (264.7215, 181.1594) (264.7992, 181.2097) (264.9001, 181.2807) (265.0226, 181.3748) (265.1426, 181.4727) (265.2609, 181.5729) (265.3784, 181.6744) (265.4954, 181.7767) (265.6117, 181.88) (265.7271, 181.9844) (265.8414, 182.0903) (265.9544, 182.1981) (266.066, 182.3077) (266.1764, 182.419) (266.2857, 182.5316) (266.3942, 182.6455) (266.5018, 182.7603) (266.6087, 182.876) (266.7148, 182.9927) (266.8201, 183.1105) (266.9246, 183.2292) (267.0281, 183.3491) (267.1308, 183.47) (267.2327, 183.5919) (267.3337, 183.7148) (267.434, 183.8386) (267.5335, 183.9633) (267.6323, 184.0888) (267.7304, 184.2151) (267.8277, 184.3423) (267.9243, 184.4703) (268.0201, 184.5991) (268.1152, 184.7288) (268.2096, 184.8592) (268.3032, 184.9905) (268.3962, 185.1224) (268.4884, 185.2552) (268.58, 185.3886) (268.6708, 185.5228) (268.761, 185.6577) (268.8505, 185.7933) (268.9393, 185.9295) (269.0275, 186.0665) (269.1149, 186.2042) (269.2017, 186.3425) (269.2878, 186.4815) (269.3733, 186.6211) (269.4581, 186.7614) (269.5422, 186.9023) (269.6257, 187.0438) (269.7085, 187.186) (269.7907, 187.3288) (269.8723, 187.4721) (269.9532, 187.6161) (270.0334, 187.7607) (270.113, 187.9058) (270.192, 188.0515) (270.2703, 188.1978) (270.348, 188.3447) (270.4251, 188.4921) (270.5015, 188.6401) (270.5773, 188.7886) (270.6525, 188.9377) (270.727, 189.0873) (270.801, 189.2374) (270.8743, 189.3881) (270.9469, 189.5393) (271.019, 189.6909) (271.0904, 189.8431) (271.1471, 189.9653) (271.1893, 190.0572) (271.2173, 190.1185) (271.2313, 190.1492) knots 0 0 0 0 0 0 0.01428571 0.02857143 0.04285714 0.05714286 0.07142857 0.08571429 0.1 0.11428571 0.12857143 0.14285714 0.15714286 0.17142857 0.18571429 0.2 0.21428571 0.22857143 0.24285714 0.25714286 0.27142857 0.28571429 0.3 0.31428571 0.32857143 0.34285714 0.35714286 0.37142857 0.38571429 0.4 0.41428571 0.42857143 0.44285714 0.45714286 0.47142857 0.48571429 0.5 0.51428571 0.52857143 0.54285714 0.55714286 0.57142857 0.58571429 0.6 0.61428571 0.62857143 0.64285714 0.65714286 0.67142857 0.68571429 0.7 0.71428571 0.72857143 0.74285714 0.75714286 0.77142857 0.78571429 0.8 0.81428571 0.82857143 0.84285714 0.85714286 0.87142857 0.88571429 0.9 0.91428571 0.92857143 0.94285714 0.95714286 0.97142857 0.98571429 1 1 1 1 1 1
  line L1289 (264.6423, 181.1115) -> (264.6688, 181.1272) construction
  line L1290 (264.6688, 181.1272) -> (264.7215, 181.1594) construction
  line L1291 (264.7215, 181.1594) -> (264.7992, 181.2097) construction
  line L1292 (264.7992, 181.2097) -> (264.9001, 181.2807) construction
  line L1293 (264.9001, 181.2807) -> (265.0226, 181.3748) construction
  line L1294 (265.0226, 181.3748) -> (265.1426, 181.4727) construction
  line L1295 (265.1426, 181.4727) -> (265.2609, 181.5729) construction
  line L1296 (265.2609, 181.5729) -> (265.3784, 181.6744) construction
  line L1297 (265.3784, 181.6744) -> (265.4954, 181.7767) construction
  line L1298 (265.4954, 181.7767) -> (265.6117, 181.88) construction
  line L1299 (265.6117, 181.88) -> (265.7271, 181.9844) construction
  line L1300 (265.7271, 181.9844) -> (265.8414, 182.0903) construction
  line L1301 (265.8414, 182.0903) -> (265.9544, 182.1981) construction
  line L1302 (265.9544, 182.1981) -> (266.066, 182.3077) construction
  line L1303 (266.066, 182.3077) -> (266.1764, 182.419) construction
  line L1304 (266.1764, 182.419) -> (266.2857, 182.5316) construction
  line L1305 (266.2857, 182.5316) -> (266.3942, 182.6455) construction
  line L1306 (266.3942, 182.6455) -> (266.5018, 182.7603) construction
  line L1307 (266.5018, 182.7603) -> (266.6087, 182.876) construction
  line L1308 (266.6087, 182.876) -> (266.7148, 182.9927) construction
  line L1309 (266.7148, 182.9927) -> (266.8201, 183.1105) construction
  line L1310 (266.8201, 183.1105) -> (266.9246, 183.2292) construction
  line L1311 (266.9246, 183.2292) -> (267.0281, 183.3491) construction
  line L1312 (267.0281, 183.3491) -> (267.1308, 183.47) construction
  line L1313 (267.1308, 183.47) -> (267.2327, 183.5919) construction
  line L1314 (267.2327, 183.5919) -> (267.3337, 183.7148) construction
  line L1315 (267.3337, 183.7148) -> (267.434, 183.8386) construction
  line L1316 (267.434, 183.8386) -> (267.5335, 183.9633) construction
  line L1317 (267.5335, 183.9633) -> (267.6323, 184.0888) construction
  line L1318 (267.6323, 184.0888) -> (267.7304, 184.2151) construction
  line L1319 (267.7304, 184.2151) -> (267.8277, 184.3423) construction
  line L1320 (267.8277, 184.3423) -> (267.9243, 184.4703) construction
  line L1321 (267.9243, 184.4703) -> (268.0201, 184.5991) construction
  line L1322 (268.0201, 184.5991) -> (268.1152, 184.7288) construction
  line L1323 (268.1152, 184.7288) -> (268.2096, 184.8592) construction
  line L1324 (268.2096, 184.8592) -> (268.3032, 184.9905) construction
  line L1325 (268.3032, 184.9905) -> (268.3962, 185.1224) construction
  line L1326 (268.3962, 185.1224) -> (268.4884, 185.2552) construction
  line L1327 (268.4884, 185.2552) -> (268.58, 185.3886) construction
  line L1328 (268.58, 185.3886) -> (268.6708, 185.5228) construction
  line L1329 (268.6708, 185.5228) -> (268.761, 185.6577) construction
  line L1330 (268.761, 185.6577) -> (268.8505, 185.7933) construction
  line L1331 (268.8505, 185.7933) -> (268.9393, 185.9295) construction
  line L1332 (268.9393, 185.9295) -> (269.0275, 186.0665) construction
  line L1333 (269.0275, 186.0665) -> (269.1149, 186.2042) construction
  line L1334 (269.1149, 186.2042) -> (269.2017, 186.3425) construction
  line L1335 (269.2017, 186.3425) -> (269.2878, 186.4815) construction
  line L1336 (269.2878, 186.4815) -> (269.3733, 186.6211) construction
  line L1337 (269.3733, 186.6211) -> (269.4581, 186.7614) construction
  line L1338 (269.4581, 186.7614) -> (269.5422, 186.9023) construction
  line L1339 (269.5422, 186.9023) -> (269.6257, 187.0438) construction
  line L1340 (269.6257, 187.0438) -> (269.7085, 187.186) construction
  line L1341 (269.7085, 187.186) -> (269.7907, 187.3288) construction
  line L1342 (269.7907, 187.3288) -> (269.8723, 187.4721) construction
  line L1343 (269.8723, 187.4721) -> (269.9532, 187.6161) construction
  line L1344 (269.9532, 187.6161) -> (270.0334, 187.7607) construction
  line L1345 (270.0334, 187.7607) -> (270.113, 187.9058) construction
  line L1346 (270.113, 187.9058) -> (270.192, 188.0515) construction
  line L1347 (270.192, 188.0515) -> (270.2703, 188.1978) construction
  line L1348 (270.2703, 188.1978) -> (270.348, 188.3447) construction
  line L1349 (270.348, 188.3447) -> (270.4251, 188.4921) construction
  line L1350 (270.4251, 188.4921) -> (270.5015, 188.6401) construction
  line L1351 (270.5015, 188.6401) -> (270.5773, 188.7886) construction
  line L1352 (270.5773, 188.7886) -> (270.6525, 188.9377) construction
  line L1353 (270.6525, 188.9377) -> (270.727, 189.0873) construction
  line L1354 (270.727, 189.0873) -> (270.801, 189.2374) construction
  line L1355 (270.801, 189.2374) -> (270.8743, 189.3881) construction
  line L1356 (270.8743, 189.3881) -> (270.9469, 189.5393) construction
  line L1357 (270.9469, 189.5393) -> (271.019, 189.6909) construction
  line L1358 (271.019, 189.6909) -> (271.0904, 189.8431) construction
  line L1359 (271.0904, 189.8431) -> (271.1471, 189.9653) construction
  line L1360 (271.1471, 189.9653) -> (271.1893, 190.0572) construction
  line L1361 (271.1893, 190.0572) -> (271.2173, 190.1185) construction
  line L1362 (271.2173, 190.1185) -> (271.2313, 190.1492) construction
  line L1363 (225.137, 92.0377) -> (225.4942, 90.4458)
  line L1364 (225.137, 92.0377) -> (225.4942, 90.4458)
  line L1365 (172.8837, 194.5906) -> (171.8057, 195.8153)
  circle A41 centre (212.132, 150) radius 2.3
  arc A42 (172.7536, 191.8132) -> (170.3188, 189.3784) centre (212.132, 150) ccw
  line L1366 (172.8837, 194.5906) -> (171.8057, 195.8153)
  arc A43 (172.7536, 191.8132) -> (170.3188, 189.3784) centre (212.132, 150) ccw
  arc A44 (172.7536, 191.8132) -> (172.8837, 194.5906) centre (171.3824, 193.2692) ccw
  arc A45 (167.5414, 189.2483) -> (170.3188, 189.3784) centre (168.8628, 190.7496) ccw
  arc A46 (172.7536, 191.8132) -> (172.8837, 194.5906) centre (171.3824, 193.2692) ccw
  circle A47 centre (212.132, 150) radius 2.3
  arc A48 (167.5414, 189.2483) -> (170.3188, 189.3784) centre (168.8628, 190.7496) ccw